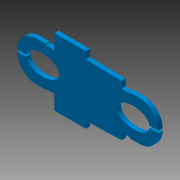
# Autodesk Inventor part: LockZ
Saved by Autodesk Inventor 2014 SP2 (Build 180246200, 246)
## iProperties
Created: 2014-11-24
Part Number: LockZ
Material: Generic
Document SubType Name: Modeling
Designer: JLM
Density: 1 g/cm^3
Appearance: Default
Author: JLM
Autodesk Inventor part; units mm, degrees
ref_plane "YZ Plane" through (0, 0, 0) normal (1, 0, 0) x (0, 1, 0)
ref_plane "XZ Plane" through (0, 0, 0) normal (0, 1, 0) x (-1, 0, 0)
ref_plane "XY Plane" through (0, 0, 0) normal (0, 0, 1) x (1, 0, 0)
sketch "Sketch1" plane through (0, 0, 0) normal (0, 0, 1) x (1, 0, 0)
  line L0 (47.1932, 0) -> (47.1932, 13.335)
  line L1 (47.1932, 13.335) -> (28.1432, 13.335)
  line L2 (28.1432, 13.335) -> (28.1432, 12.6365)
  line L3 (28.1432, 12.6365) -> (22.4282, 12.6365)
  line L4 (12.2521, 0) -> (47.1932, 0)
  line L5 (22.4282, 12.6365) -> (22.4282, 22.4282)
  line L6 (22.4282, 22.4282) -> (0, 22.4282)
  line L7 (47.1932, 0.762) -> (41.2045, 0.762)
  line L8 (47.1932, 0) -> (47.1932, -13.335)
  line L9 (47.1932, -13.335) -> (28.1432, -13.335)
  line L10 (28.1432, -13.335) -> (28.1432, -12.6365)
  line L11 (28.1432, -12.6365) -> (22.4282, -12.6365)
  line L12 (22.4282, -12.6365) -> (22.4282, -22.4282)
  line L13 (22.4282, -22.4282) -> (0, -22.4282)
  line L14 (47.1932, -0.762) -> (41.2045, -0.762)
  line L15 (0, 22.4282) -> (0, -22.4282)
  ellipse E0 centre (30.2836, 0) end of major axis (41.275, 0) minor radius 6.7381 (41.2045, 0.762) -> (41.2045, -0.762) ccw
  point P0 (0, 0)
  point P1 (17.8114, 0)
  point P2 (41.275, 0.762)
  point P3 (41.275, -0.762)
  dimension "d0" = 13.335
  dimension "d1" = 19.05
  dimension "d6" = 12.6365
  dimension "d7" = 22.4282
  dimension "d8" = 22.4282
  dimension "d9" = 5.715
  dimension "d16" = 44.8564
  dimension "d17" = 47.1932
  dimension "d34" = 0.762
  constraints: 32 end point, 8 symmetric about line, 7 point on line, 4 perpendicular, 2 parallel, 4 other
  measures "d0" distance of L0.start L0.end
  measures "d1" distance of L0.end L1.end
  measures "d6" distance between parallel lines of L4 L3
  measures "d7" distance between parallel lines of L4 L6
  measures "d8" distance from line of L5 point (0, 0)
  measures "d9" distance of L2.end L3.end
  measures "d16" distance between parallel lines of L13 L6
  measures "d17" distance from line of L8 point (0, 0)
  measures "d34" distance between parallel lines of L4 L7
extrude "Extrusion2" add sketch "Sketch1" along normal blind 2.794 contours L7 E0 L14 L8 L9 L10 L11 L12 L13 L15 L6 L5 L3 L2 L1 L0
pattern_circular "Circular Pattern1" count 2 over 360 about axis through (0, 0, -10) along (0, 0, 1) of "Extrusion2"
fillet "Fillet2" radius 12.7 2 edges at (47.1932, 13.335, 1.397) (47.1932, -13.335, 1.397)
fillet "Fillet3" radius 12.7 2 edges at (-47.1932, -13.335, 1.397) (-47.1932, 13.335, 1.397)
sketch "Sketch3" plane through (0, 0, 2.794) normal (0, 0, 1) x (1, 0, 0)
  line L0 (22.4282, 12.6365) -> (22.4282, 22.4282) projected
  line L1 (22.4282, 22.4282) -> (-22.4282, 22.4282) projected
  line L2 (-1.397, 17.78) -> (22.4282, 17.1287)
  line L3 (22.4282, 22.4282) -> (22.4282, 17.1287)
  line L4 (0, 0) -> (6.35, 0)
  line L5 (22.4282, -12.6365) -> (22.4282, -22.4282)
  line L6 (22.4282, -22.4282) -> (22.4282, -17.1287)
  line L7 (-28.1432, 13.335) -> (-34.4938, 13.335) projected
  line L8 (-1.397, 22.4282) -> (-1.397, 17.78)
  line L9 (22.0067, 22.4282) -> (-1.397, 22.4282)
  line L10 (22.4282, -12.6365) -> (22.4282, -22.4282)
  line L11 (22.4282, -22.4282) -> (-22.4282, -22.4282)
  line L12 (-1.397, -17.78) -> (22.4282, -17.1287)
  line L13 (-1.397, -22.4282) -> (-1.397, -17.78)
  point P0 (0, 22.4282)
  dimension "d32" = 1.397
  dimension "d33" = 17.78
  constraints: 22 end point, 6 point on line, 3 perpendicular, 3 symmetric about line, 1 collinear, 1 midpoint
  measures "d32" distance from line of L4.start L8
  measures "d33" vertical distance of L4.start L2.start
extrude "Extrusion4" cut sketch "Sketch3" against normal up to next
equation "\"d7\" = d8"
body "Solid2"
